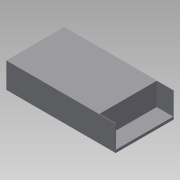
# Autodesk Inventor part: powersupply
Saved by Autodesk Inventor 2015 (Build 190159000, 159)
## iProperties
Created: 2015-05-21
Part Number: powersupply
Material: Generic
Document SubType Name: Modeling
Designer: Joe Sheldon
Density: 1 g/cm^3
Appearance: Default
Author: Joe Sheldon
Autodesk Inventor part; units mm, degrees
ref_plane "YZ Plane" through (0, 0, 0) normal (1, 0, 0) x (0, 1, 0)
ref_plane "XZ Plane" through (0, 0, 0) normal (0, 1, 0) x (-1, 0, 0)
ref_plane "XY Plane" through (0, 0, 0) normal (0, 0, 1) x (1, 0, 0)
sketch "Sketch1" plane through (0, 0, 0) normal (0, 1, 0) x (-1, 0, 0)
  line L0 (0, 0) -> (215, 0)
  line L1 (215, 0) -> (215, -114)
  line L2 (215, -114) -> (0, -114)
  line L3 (0, -114) -> (0, 0)
  dimension "d0" = 215
  dimension "d1" = 114
  constraints: 8 end point, 2 parallel, 1 horizontal, 1 perpendicular
  measures "d0" distance of L1.end L2.end
  measures "d1" distance of L0.end L1.end
extrude "Extrusion1" add sketch "Sketch1" along normal blind 50
sketch "Sketch2" plane through (0, 0, 0) normal (1, 0, 0) x (0, 0, -1)
  line L0 (0, 50) -> (114, 50) projected
  line L1 (0.7711, 50) -> (113.1846, 50)
  line L2 (113.1846, 50) -> (113.1846, 5.3407)
  line L3 (113.1846, 5.3407) -> (0.7711, 5.3407)
  line L4 (0.7711, 5.3407) -> (0.7711, 50)
  point P0 (0, 0)
  constraints: 8 end point, 2 parallel, 1 horizontal, 1 perpendicular, 1 point on line
extrude "Extrusion2" cut sketch "Sketch2" against normal blind 32.55
body "Solid1"
